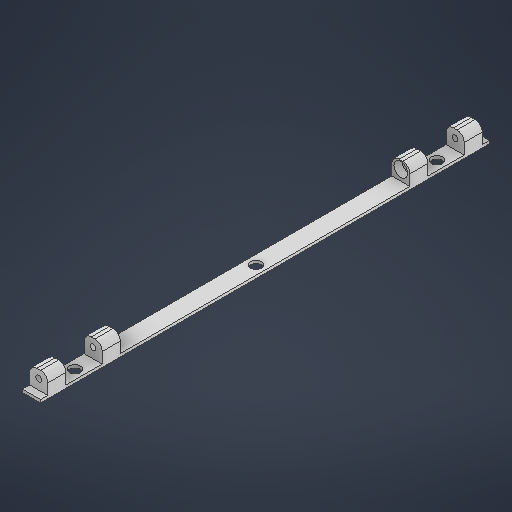
# Autodesk Inventor part: zawiasv2
Saved by Autodesk Inventor 2026.2 (Build 302298010, 298A)
## iProperties
Created: 2026-05-22
Part Number: zawiasv2
Material: Ogólny
Document SubType Name: Modeling
Designer: karol
Density: 1 g/cm^3
Appearance: Domyślna
Author: karol
Autodesk Inventor part; units mm, degrees
ref_plane "YZ Plane" through (0, 0, 0) normal (1, 0, 0) x (0, 1, 0)
ref_plane "XZ Plane" through (0, 0, 0) normal (0, 1, 0) x (-1, 0, 0)
ref_plane "XY Plane" through (0, 0, 0) normal (0, 0, 1) x (1, 0, 0)
sketch "Szkic1" plane through (0, 0, 0) normal (0, 1, 0) x (-1, 0, 0)
  line L0 (0, 0) -> (5, 0)
  line L1 (5, 0) -> (5, -62)
  line L2 (5, -62) -> (0, -62)
  line L3 (0, -62) -> (0, 0)
  line L4 (0, 0) -> (5, 0)
  line L5 (5, 0) -> (5, 62)
  line L6 (5, 62) -> (0, 62)
  line L7 (0, 62) -> (0, 0)
  line L8 (0, 62) -> (5, 62)
  line L9 (5, 62) -> (5, 60)
  line L10 (5, 60) -> (0, 60)
  line L11 (0, 60) -> (0, 62)
  line L12 (5, 60) -> (0, 60)
  line L13 (0, 60) -> (0, 55)
  line L14 (0, 55) -> (5, 55)
  line L15 (5, 55) -> (5, 60)
  line L16 (5, 55) -> (0, 55)
  line L17 (0, 55) -> (0, 45)
  line L18 (0, 45) -> (5, 45)
  line L19 (5, 45) -> (5, 55)
  line L20 (5, 45) -> (0, 45)
  line L21 (0, 45) -> (0, 40)
  line L22 (0, 40) -> (5, 40)
  line L23 (5, 40) -> (5, 45)
  line L24 (0, 40) -> (5, 40)
  line L25 (5, 40) -> (5, 38)
  line L26 (5, 38) -> (0, 38)
  line L27 (0, 38) -> (0, 40)
  line L28 (0, -62) -> (5, -62)
  line L29 (5, -62) -> (5, -60)
  line L30 (5, -60) -> (0, -60)
  line L31 (0, -60) -> (0, -62)
  line L32 (0, -60) -> (5, -60)
  line L33 (5, -60) -> (5, -55)
  line L34 (5, -55) -> (0, -55)
  line L35 (0, -55) -> (0, -60)
  line L36 (0, -55) -> (5, -55)
  line L37 (5, -55) -> (5, -45)
  line L38 (5, -45) -> (0, -45)
  line L39 (0, -45) -> (0, -55)
  line L40 (0, -45) -> (5, -45)
  line L41 (5, -45) -> (5, -40)
  line L42 (5, -40) -> (0, -40)
  line L43 (0, -40) -> (0, -45)
  line L44 (0, -40) -> (5, -40)
  line L45 (5, -40) -> (5, -38)
  line L46 (5, -38) -> (0, -38)
  line L47 (0, -38) -> (0, -40)
  point P0 (0, -45)
  point P1 (0, -55)
  point P2 (5, 40)
  point P3 (5, 55)
  point P4 (0, 60)
  dimension "d0" = 5
  dimension "d1" = 62
  dimension "d2" = 62
  dimension "d3" = 2
  dimension "d4" = 5
  dimension "d5" = 10
  dimension "d6" = 5
  dimension "d7" = 2
  dimension "d8" = 2
  dimension "d9" = 5
  dimension "d10" = 10
  dimension "d11" = 5
  dimension "d12" = 2
  constraints: 96 end point, 24 parallel, 12 horizontal, 12 perpendicular, 11 point on line
  measures "d0" distance of L1.end L2.end
  measures "d1" distance of L0.end L1.end
  measures "d2" distance of L5.end L4.end
  measures "d3" distance of L8.end L9.end
  measures "d4" distance of L13.end L12.end
  measures "d5" distance of L17.end L16.end
  measures "d6" distance of L21.end L20.end
  measures "d7" distance of L24.end L25.end
  measures "d8" distance of L29.end L28.end
  measures "d9" distance of L33.end L32.end
  measures "d10" distance of L37.end L36.end
  measures "d11" distance of L41.end L40.end
  measures "d12" distance of L45.end L44.end
extrude "Wyciągnięcie proste1" add sketch "Szkic1" against normal blind 0.8
extrude "Wyciągnięcie proste2" add sketch "Szkic1" along normal blind 5 contours L42 L1 L38 L3 | L7 L18 L5 L22 | L34 L1 L30 L3 | L7 L10 L5 L14
sketch "Szkic2" plane through (0, 0, 40) normal (0, 0, -1) x (-1, 0, 0)
  circle A0 centre (2.5, 2.8) radius 1.9
  circle A1 centre (2.5, 2.8) radius 0.8
  line L0 (5, 0) -> (5, 5) projected
  line L1 (0, 5) -> (5, 5) projected
  point P0 (0, 0)
  point P1 (5, 2.5)
  dimension "d17" = 3.8
  dimension "d18" = 1.6
  dimension "d19" = 2.5
  dimension "d20" = 2.2
  constraints: 2 centre point, 1 coincident, 1 midpoint
  measures "d17" diameter of A0
  measures "d18" diameter of A1
  measures "d19" horizontal distance of point (5, 2.5) A0.centre
  measures "d20" distance from line of L1 A0.centre
extrude "Wyciągnięcie proste3" cut sketch "Szkic2" against normal blind 2.2 contours A0 | A1
extrude "Wyciągnięcie proste4" cut sketch "Szkic2" against normal blind 20 contours A1
thread "Gwint1" size "M2x0.4" class "6H" standard "ANSI Metric M Profile" full length
sketch "Szkic3" plane through (-5, 0, -40) normal (0, 0, 1) x (1, 0, 0)
  circle A0 centre (2.5, 2.8) radius 0.8 projected
  circle A1 centre (2.5, 2.8) radius 1.9
  circle A2 centre (2.5, 2.8) radius 0.8
  point P0 (5, 0)
  dimension "d27" = 3.8
  dimension "d28" = 1.6
  constraints: 2 centre point, 2 coincident
  measures "d27" diameter of A1
  measures "d28" diameter of A2
extrude "Wyciągnięcie proste5" cut sketch "Szkic3" against normal blind 2.2 contours A0 | A1
extrude "Wyciągnięcie proste6" cut sketch "Szkic3" against normal blind 20 contours A0
thread "Gwint2" size "M2x0.4" class "6H" standard "ANSI Metric M Profile" full length
fillet "Zaokrąglenie1" radius 2 8 edges at (-5, 5, 57.5) (0, 5, 57.5) (0, 5, 42.5) (-5, 5, 42.5) (0, 5, -42.5) (-5, 5, -42.5) (0, 5, -57.5) (-5, 5, -57.5)
sketch "Szkic4" plane through (0, 0, 0) normal (0, 1, 0) x (1, 0, 0)
  circle A0 centre (-2.5, -50) radius 1.55
  circle A1 centre (-2.5, 50) radius 1.55
  circle A2 centre (-2.5, 0) radius 1.55
  line L0 (-5, -45) -> (-5, -55) projected
  line L1 (-3, -45) -> (-2, -45) projected
  line L2 (-2, 45) -> (-3, 45) projected
  line L3 (-5, 55) -> (-5, 45) projected
  line L4 (-5, 40) -> (-5, -40) projected
  line L5 (0, 62) -> (-5, 62) projected
  point P0 (0, 0)
  point P1 (-2.5, -45)
  point P2 (-2.5, 45)
  point P3 (-5, 50)
  point P4 (-2.5, 62)
  dimension "d36" = 3.1
  dimension "d37" = 2.5
  dimension "d38" = 5
  dimension "d39" = 5
  dimension "d40" = 2.5
  dimension "d41" = 3.1
  dimension "d42" = 2.5
  dimension "d43" = 62
  dimension "d44" = 3.1
  constraints: 4 midpoint, 3 centre point
  measures "d36" diameter of A0
  measures "d37" distance from line of L0 A0.centre
  measures "d38" distance of point (-2.5, -45) A0.centre
  measures "d39" distance of point (-2.5, 45) A1.centre
  measures "d40" distance of point (-5, 50) A1.centre
  measures "d41" diameter of A1
  measures "d42" distance from line of L4 A2.centre
  measures "d43" distance of point (-2.5, 62) A2.centre
  measures "d44" diameter of A2
extrude "Wyciągnięcie proste7" cut sketch "Szkic4" against normal blind 0.8
